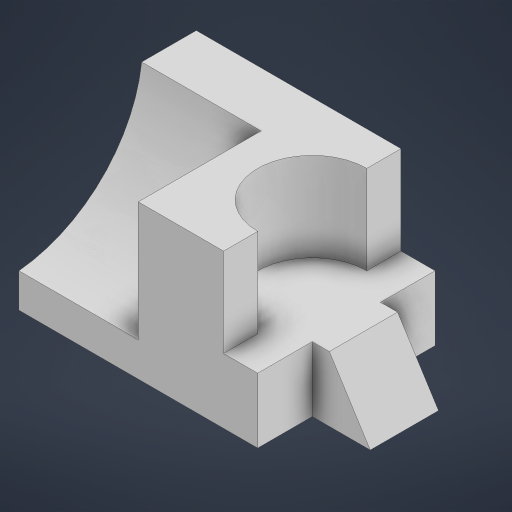
# Autodesk Inventor part: Part1
Saved by Autodesk Inventor 2024 (Build 280153000, 153)
## iProperties
Created: 2024-02-24
Part Number: Part1
Material: Generic
Document SubType Name: Modeling
Designer: Papryk
Density: 1 g/cm^3
Appearance: Default
Author: Papryk
Autodesk Inventor part; units mm, degrees
ref_plane "YZ Plane" through (0, 0, 0) normal (1, 0, 0) x (0, 1, 0)
ref_plane "XZ Plane" through (0, 0, 0) normal (0, 1, 0) x (-1, 0, 0)
ref_plane "XY Plane" through (0, 0, 0) normal (0, 0, 1) x (1, 0, 0)
sketch "Sketch1" plane through (0, 0, 0) normal (0, 1, 0) x (-1, 0, 0)
  line L0 (0, 0) -> (25, 0)
  line L1 (25, 0) -> (25, 52)
  line L2 (25, 52) -> (0, 52)
  line L3 (0, 52) -> (0, 42)
  line L4 (0, 0) -> (0, 10)
  arc A0 (0, 10) -> (0, 42) centre (0, 26) ccw
  dimension "d0" = 25
  dimension "d1" = 52
  dimension "d3" = 10
  dimension "d4" = 10
  dimension "d5" = 16
  constraints: 10 end point, 2 point on circle, 2 vertical, 1 centre point, 1 horizontal, 1 parallel, 1 perpendicular
  measures "d0" distance of L2.end L1.end
  measures "d1" distance of L1.end L0.end
  measures "d3" distance of L2.end L3.end
  measures "d4" distance of L0.start L4.end
  measures "d5" radius of A0
extrude "Extrusion1" add sketch "Sketch1" along normal blind 26
sketch "Sketch2" plane through (-25, 0, 0) normal (-1, 0, 0) x (0, 0, 1)
  line L0 (0, 26) -> (0, -19)
  line L1 (0, -19) -> (52, -19)
  line L2 (52, -19) -> (52, -9)
  line L3 (0, 26) -> (16, 26)
  line L4 (0, 26) -> (52, 26) projected
  arc A0 (16, 26) -> (52, -9) centre (55.7076, 30.8278) ccw
  point P0 (0, 0)
  dimension "d8" = 45
  dimension "d9" = 52
  dimension "d10" = 90
  dimension "d11" = 10
  dimension "d12" = 90
  dimension "d13" = 16
  dimension "d17" = 40
  constraints: 8 end point, 2 perpendicular, 2 point on circle, 1 centre point, 1 point on line, 1 vertical
  measures "d8" distance of L0.start L0.end
  measures "d9" distance of L0.end L1.end
  measures "d10" angle of L1 L0
  measures "d11" distance of L1.end L2.end
  measures "d12" angle of L2 L1
  measures "d13" distance of L0.start L3.end
  measures "d17" radius of A0
extrude "Extrusion2" add sketch "Sketch2" along normal blind 35
sketch "Sketch3" plane through (0, 0, 0) normal (0, -1, 0) x (1, 0, 0)
  line L0 (-25, 0) -> (-25, 30.2194) projected
  line L1 (-25, 0) -> (10, 0)
  line L2 (10, 52) -> (-25, 52)
  line L3 (-25, 52) -> (-25, 0)
  line L4 (10, 0) -> (10, 16)
  line L5 (10, 52) -> (10, 36)
  line L6 (10, 16) -> (15, 16)
  line L7 (15, 16) -> (15, 36)
  line L8 (15, 36) -> (10, 36)
  line L9 (10, 36) -> (10, 16)
  point P0 (0, 0)
  point P1 (10, 36)
  dimension "d18" = 35
  dimension "d19" = 16
  dimension "d20" = 16
  dimension "d21" = 5
  dimension "d27" = 35
  constraints: 18 end point, 3 parallel, 2 horizontal, 2 vertical, 1 perpendicular
  measures "d18" distance of L2.end L2.start
  measures "d19" distance of L1.end L4.end
  measures "d20" distance of L2.start L5.end
  measures "d21" distance of L8.end L7.end
  measures "d27" distance of L0.start L1.end
extrude "Extrusion3" add sketch "Sketch3" along normal blind 19
sketch "Sketch4" plane through (10, 0, 36) normal (0, 0, 1) x (1, 0, 0)
  line L0 (5, 0) -> (5, -19) projected
  line L1 (5, -19) -> (17, -19)
  line L2 (17, -19) -> (5, 0)
  line L3 (5, 0) -> (5, -19)
  point P0 (-10, 0)
  dimension "d24" = 12
  constraints: 6 end point, 1 collinear, 1 horizontal
  measures "d24" distance of L0.end L1.end
extrude "Extrusion4" add sketch "Sketch4" against normal blind 20
equation "\"d20\" = d19"
equation "\"d27\" = d18"
body "Solid1"
